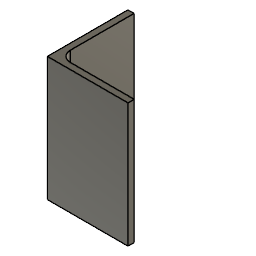
L-65×65×5 (Autodesk Fusion 360 design; units mm, degrees)
Autodesk Fusion 360 part; units mm, degrees
note: some values were not read from the file. Set by a fixed rule: which sketch regions a step uses.
sketch "スケッチ1" plane through (0, 0, 0) normal (0, 0, 1) x (1, 0, 0)
  line L0 (0, 65) -> (0, 0)
  line L1 (5, 13.5) -> (5, 65)
  line L2 (65, 5) -> (13.5, 5)
  line L3 (0, 0) -> (65, 0)
  arc A0 (5, 13.5) -> (13.5, 5) centre (13.5, 13.5) ccw
  line L4 (65, 0) -> (65, 5)
  line L5 (5, 65) -> (0, 65)
extrude "押し出し1" add sketch "スケッチ1" along normal blind 100
